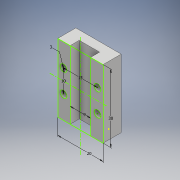
# Autodesk Inventor part: slider-slider
Saved by Autodesk Inventor 2018 (Build 220112000, 112)
## iProperties
Created: 2025-02-27
Part Number: slider-slider
Material: Generic
Document SubType Name: Modeling
Designer: neo
Density: 1 g/cm^3
Appearance: Default
Author: neo
Autodesk Inventor part; units mm, degrees
ref_plane "YZ Plane" through (0, 0, 0) normal (1, 0, 0) x (0, 1, 0)
ref_plane "XZ Plane" through (0, 0, 0) normal (0, 1, 0) x (-1, 0, 0)
ref_plane "XY Plane" through (0, 0, 0) normal (0, 0, 1) x (1, 0, 0)
sketch "Sketch1" plane through (0, 0, 0) normal (0, 1, 0) x (-1, 0, 0)
  line L0 (22.5467, 23.3874) -> (2.5467, 23.3874)
  line L1 (2.5467, 23.3874) -> (2.5467, -6.6126)
  line L2 (2.5467, -6.6126) -> (22.5467, -6.6126)
  line L3 (22.5467, -6.6126) -> (22.5467, 23.3874)
  line L4 (12.5467, -16.022) -> (12.5467, 29.6209)
  line L5 (17.0467, 23.3874) -> (8.0467, 23.3874)
  line L6 (8.0467, 23.3874) -> (8.0467, -6.6126)
  line L7 (8.0467, -6.6126) -> (17.0467, -6.6126)
  line L8 (17.0467, -6.6126) -> (17.0467, 23.3874)
  line L9 (26.0194, 8.3874) -> (1.0659, 8.3874)
  circle A0 centre (20.0467, 13.3874) radius 1.5
  circle A1 centre (5.0467, 13.3874) radius 1.5
  circle A2 centre (20.0467, 3.3874) radius 1.5
  circle A3 centre (5.0467, 3.3874) radius 1.5
  point P0 (0, 0)
  dimension "WR" = 9
  dimension "L" = 30
  dimension "d3" = 20
  dimension "d4" = 3
  dimension "d7" = 15
  dimension "d10" = 10
  constraints: 20 end point, 4 centre point, 4 horizontal, 4 parallel, 2 perpendicular, 2 point on line, 2 vertical, 11 other
  measures "WR" distance between parallel lines of L6 L8
  measures "L" distance of L0.end L1.end
  measures "d3" distance between parallel lines of L1 L3
  measures "d4" diameter of A0
  measures "d7" distance of A0.centre A1.centre
  measures "d10" distance of A0.centre A2.centre
extrude "Extrusion1" add sketch "Sketch1" along normal blind 8
extrude "Extrusion2" cut sketch "Sketch1" along normal blind 4 contours L8 L9 L4 L0 | L4 L9 L6 L0 | L8 L2 L4 L9 | L4 L2 L6 L9
body "Solid1"
